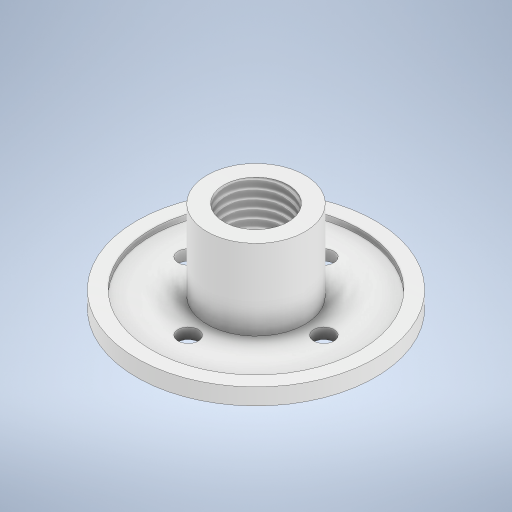
# Autodesk Inventor part: Flanche
Saved by Autodesk Inventor 2024 (Build 280153000, 153)
## iProperties
Created: 2022-09-01
Part Number: Flanche
Material: PVC, no plastificado
Document SubType Name: Modeling
Designer: Usuario
Density: 1.29 g/cm^3
Appearance: Suave - Blanco
Mass: 28.1107 g
Surface Area: 123.487 cm^2
Volume: 21.7912 cm^3
Author: Usuario
Autodesk Inventor part; units mm, degrees
ref_plane "YZ Plane" through (0, 0, 0) normal (1, 0, 0) x (0, 1, 0)
ref_plane "XZ Plane" through (0, 0, 0) normal (0, 1, 0) x (-1, 0, 0)
ref_plane "XY Plane" through (0, 0, 0) normal (0, 0, 1) x (1, 0, 0)
sketch "Boceto1" plane through (0, 0, 0) normal (0, 1, 0) x (-1, 0, 0)
  circle A0 centre (0, 0) radius 35.165
  circle A1 centre (0, 0) radius 9.485
  circle A2 centre (0, 0) radius 14.45
  dimension "d0" = 70.33
  dimension "d23" = 18.97
  dimension "d24" = 28.9
  constraints: 3 centre point, 3 coincident
  measures "d0" diameter of A0
  measures "d23" diameter of A1
  measures "d24" diameter of A2
extrude "Extrusión1" add sketch "Boceto1" along normal blind 26.85 contours A2
extrude "Extrusión2" add sketch "Boceto1" along normal blind 4.85 contours A0
thread "Rosca1" size "M20x2.5" class "6H" standard "ANSI Metric M Profile" full length
sketch "Boceto2" plane through (0, 4.85, 0) normal (0, 1, 0) x (1, 0, 0)
  circle A0 centre (0, 0) radius 30.835
  dimension "d9" = 61.67
  constraints: 1 centre point, 1 coincident
  measures "d9" diameter of A0
extrude "Extrusión3" cut sketch "Boceto2" against normal blind 1.67
sketch "Boceto3" plane through (0, 4.85, 0) normal (0, -1, 0) x (1, 0, 0)
  circle A0 centre (0, 0) radius 14.45 projected
  circle A1 centre (0, 0) radius 9.485 projected
extrude "Extrusión4" add sketch "Boceto3" along normal through all
sketch "Boceto4" plane through (0, 0, 0) normal (0, -1, 0) x (1, 0, 0)
  circle A0 centre (-20, 0) radius 3
  circle A1 centre (0, -20) radius 3
  circle A2 centre (20, 0) radius 3
  circle A3 centre (0, 20) radius 3
  point P0 (0, 0)
  dimension "d14" = 6
  dimension "d15" = 20
  dimension "d16" = 0
  dimension "d19" = 360
  constraints: 4 centre point, 9 other
  measures "d14" diameter of A0
  measures "d15" distance of point (0, 0) A0.centre
  measures "d16" vertical distance of point (0, 0) A0.centre
extrude "Extrusión5" cut sketch "Boceto4" against normal blind 26.85
